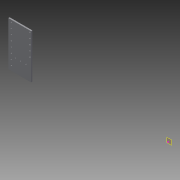
# Autodesk Inventor part: Aluminum Mounting Plate
Saved by Autodesk Inventor 2015 (Build 190159000, 159)
## iProperties
Created: 2015-01-27
Part Number: Aluminum Mounting Plate
Material: Generic
Document SubType Name: Modeling
Designer: jhirshland1
Density: 1 g/cm^3
Appearance: Default
Author: jhirshland1
Autodesk Inventor part; units mm, degrees
ref_plane "YZ Plane" through (0, 0, 0) normal (1, 0, 0) x (0, 1, 0)
ref_plane "XZ Plane" through (0, 0, 0) normal (0, 1, 0) x (-1, 0, 0)
ref_plane "XY Plane" through (0, 0, 0) normal (0, 0, 1) x (1, 0, 0)
ref_plane "Work Plane3" through (0, 0, 0) normal (0, 0, 1) x (1, 0, 0)
sketch "Sketch1" plane through (0, 0, 0) normal (0, 0, 1) x (1, 0, 0)
  line L0 (-755.65, -71.0123) -> (-755.65, -75.0128) projected
  line L1 (-57.15, -75.0128) -> (-755.65, -75.0128) projected
  line L2 (-57.15, -75.0128) -> (-57.15, -71.0123) projected
  line L3 (-57.15, -71.0123) -> (-755.65, -71.0123) projected
  line L4 (-57.15, -78.9498) -> (-755.65, -78.9498) projected
  line L5 (-755.65, -78.9498) -> (-647.9579, -78.9498)
  line L6 (-647.9579, -78.9498) -> (-647.9579, 130.9029)
  line L7 (-647.9579, 130.9029) -> (-755.65, 130.9029)
  line L8 (-755.65, 130.9029) -> (-755.65, -78.9498)
  point P0 (0, 0)
  constraints: 8 end point, 2 parallel, 1 horizontal, 1 perpendicular
extrude "Extrusion1" add sketch "Sketch1" along normal blind 6.35 contours L3 L6 L1 L0 | L8 L7 L6 L3 | L1 L6 L4 L8
sketch "Sketch3" plane through (0, 0, 6.35) normal (0, 0, 1) x (1, 0, 0)
  point P0 (0, 0)
sketch "Sketch4" plane through (0, 0, 6.35) normal (0, 0, 1) x (1, 0, 0)
  circle A0 centre (-654.685, 22.86) radius 3.3528 projected
  circle A1 centre (-654.685, 48.26) radius 3.3528 projected
  circle A2 centre (-654.685, 73.66) radius 3.3528 projected
  circle A3 centre (-654.685, 99.06) radius 3.3528 projected
  circle A4 centre (-654.685, 124.46) radius 3.3528 projected
  line L0 (-663.448, 15.875) -> (-648.335, 15.875) construction
  line L1 (-648.335, 133.985) -> (-648.335, 15.875) construction
  line L2 (-648.335, 133.985) -> (-651.51, 137.16) construction
  line L3 (-663.448, 137.16) -> (-651.51, 137.16) construction
  line L4 (-663.448, 137.16) -> (-663.448, 15.875) construction
  line L5 (-663.448, 137.16) -> (-663.448, 15.875) projected
  point P0 (0, 0)
extrude "Extrusion2" cut sketch "Sketch4" against normal blind 6.35
sketch "Sketch5" plane through (0, 0, 6.35) normal (0, 0, 1) x (1, 0, 0)
  line L0 (-736.6, -3.937) -> (-736.6, -22.225) projected
  line L1 (-460.375, -22.225) -> (-736.6, -22.225) projected
  line L2 (-460.375, -22.225) -> (-457.2, -19.05) projected
  line L3 (-457.2, -3.937) -> (-457.2, -19.05) projected
  line L4 (-736.6, -3.937) -> (-457.2, -3.937) projected
  circle A0 centre (-469.9, -15.875) radius 2.667 projected
  circle A1 centre (-495.3, -15.875) radius 2.667 projected
  circle A2 centre (-520.7, -15.875) radius 2.667 projected
  circle A3 centre (-546.1, -15.875) radius 2.667 projected
  circle A4 centre (-571.5, -15.875) radius 2.667 projected
  circle A5 centre (-596.9, -15.875) radius 2.667 projected
  circle A6 centre (-622.3, -15.875) radius 2.667 projected
  circle A7 centre (-647.7, -15.875) radius 2.667 projected
  circle A8 centre (-673.1, -15.875) radius 2.667 projected
  circle A9 centre (-698.5, -15.875) radius 2.667 projected
  circle A10 centre (-723.9, -15.875) radius 2.667 projected
  circle A11 centre (-742.95, 476.947) radius 2.667 projected
  circle A12 centre (-742.95, 451.547) radius 2.667 projected
  circle A13 centre (-742.95, 426.147) radius 2.667 projected
  circle A14 centre (-742.95, 400.747) radius 2.667 projected
  circle A15 centre (-742.95, 375.347) radius 2.667 projected
  circle A16 centre (-742.95, 349.947) radius 2.667 projected
  circle A17 centre (-742.95, 324.547) radius 2.667 projected
  circle A18 centre (-742.95, 299.147) radius 2.667 projected
  circle A19 centre (-742.95, 273.747) radius 2.667 projected
  circle A20 centre (-742.95, 248.347) radius 2.667 projected
  circle A21 centre (-742.95, 222.947) radius 2.667 projected
  circle A22 centre (-742.95, 197.547) radius 2.667 projected
  circle A23 centre (-742.95, 172.147) radius 2.667 projected
  circle A24 centre (-742.95, 146.747) radius 2.667 projected
  circle A25 centre (-742.95, 121.347) radius 2.667 projected
  circle A26 centre (-742.95, 95.947) radius 2.667 projected
  circle A27 centre (-742.95, 70.547) radius 2.667 projected
  circle A28 centre (-742.95, 45.147) radius 2.667 projected
  circle A29 centre (-742.95, 19.747) radius 2.667 projected
  circle A30 centre (-742.95, -5.653) radius 2.667 projected
  circle A31 centre (-742.95, -31.053) radius 2.667 projected
  circle A32 centre (-742.95, -56.453) radius 2.667 projected
  line L5 (-736.6, 496.0909) -> (-751.713, 496.0909) projected
  line L6 (-751.713, -75.5081) -> (-751.713, 496.0909) projected
  line L7 (-751.713, -75.5081) -> (-736.6, -75.5081) projected
  line L8 (-736.6, 496.0909) -> (-736.6, -75.5081) projected
  point P0 (0, 0)
extrude "Extrusion3" cut sketch "Sketch5" against normal blind 6.35 contours A8 | A9 | A10 | A25 | A26 | A27 | A28 | A29 | A30 | A31 | A32
body "Solid1"
